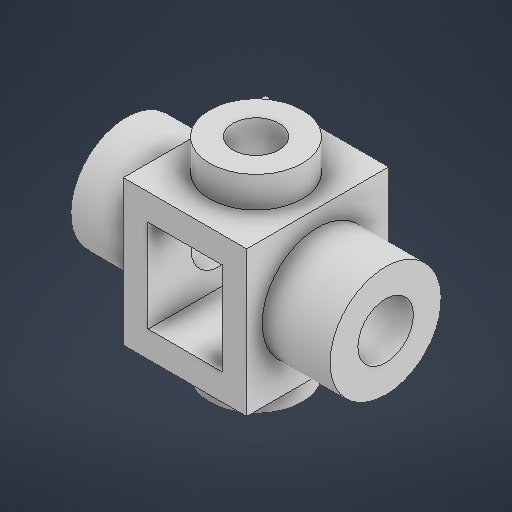
# Autodesk Inventor part: DP816
Saved by Autodesk Inventor 2025.4 (Build 294407000, 407)
## iProperties
Created: 2026-05-07
Part Number: DP816
Material: Generic
Document SubType Name: Modeling
Designer: VuQuan
Density: 1 g/cm^3
Appearance: Default
Author: VuQuan
Autodesk Inventor part; units mm, degrees
ref_plane "YZ Plane" through (0, 0, 0) normal (1, 0, 0) x (0, 1, 0)
ref_plane "XZ Plane" through (0, 0, 0) normal (0, 1, 0) x (-1, 0, 0)
ref_plane "XY Plane" through (0, 0, 0) normal (0, 0, 1) x (1, 0, 0)
sketch "Sketch1" plane through (0, 0, 0) normal (0, 0, 1) x (1, 0, 0)
  line L0 (-20, 23.5) -> (20, 23.5)
  line L1 (20, 23.5) -> (20, -23.5)
  line L2 (20, -23.5) -> (-20, -23.5)
  line L3 (-20, -23.5) -> (-20, 23.5)
  line L4 (-12, 15) -> (12, 15)
  line L5 (12, 15) -> (12, -15)
  line L6 (12, -15) -> (-12, -15)
  line L7 (-12, -15) -> (-12, 15)
  point P0 (0, 0)
  point P1 (20, 0)
  point P2 (0, 23.5)
  point P3 (12, 0)
  point P4 (0, 15)
  dimension "d0" = 40
  dimension "d1" = 47
  dimension "d2" = 24
  dimension "d12" = 30
  constraints: 16 end point, 5 parallel, 4 midpoint, 2 horizontal alignment, 2 vertical alignment, 1 horizontal, 1 perpendicular
  measures "d0" distance of L1.end L2.end
  measures "d1" distance of L0.end L1.end
  measures "d2" distance between parallel lines of L7 L5
  measures "d12" distance of L4.end L5.end
extrude "Extrusion1" add sketch "Sketch1" along normal mid plane 46
sketch "Sketch2" plane through (0, 0, 0) normal (1, 0, 0) x (0, 1, 0)
  circle A0 centre (0, 0) radius 9
  circle A1 centre (0, 0) radius 18
  dimension "d5" = 18
  dimension "d6" = 36
  constraints: 2 centre point, 2 coincident
  measures "d5" diameter of A0
  measures "d6" diameter of A1
extrude "Extrusion2" cut sketch "Sketch2" along normal through all both and the other way through all contours A0
extrude "Extrusion3" add sketch "Sketch2" along normal blind 22 from surface at 20
mirror "Mirror1" about plane through (0, 0, 0) normal (1, 0, 0) of "Extrusion3"
sketch "Sketch3" plane through (-20, 23.5, 23) normal (0, 1, 0) x (1, 0, 0)
  circle A0 centre (20, 23) radius 7.5
  circle A1 centre (20, 23) radius 15
  dimension "d13" = 15
  dimension "d14" = 30
  constraints: 3 coincident, 2 centre point
  measures "d13" diameter of A0
  measures "d14" diameter of A1
extrude "Extrusion4" cut sketch "Sketch3" against normal through all contours A0
extrude "Extrusion5" add sketch "Sketch3" along normal blind 10
mirror "Mirror2" about plane through (0, 0, 0) normal (0, 1, 0) of "Extrusion5"
ref_plane "Work Plane1" through (0, 0, 0) normal (0, 1, 0) x (-1, 0, 0)
body "Solid1"
